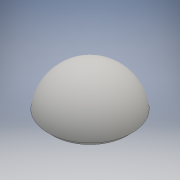
# Autodesk Inventor part: Part2
Saved by Autodesk Inventor 2016 (Build 200138000, 138)
## iProperties
Created: 2016-05-04
Part Number: Part2
Material: 一般
Document SubType Name: Modeling
Designer: 宏太
Density: 1 g/cm^3
Appearance: 既定
Author: 宏太
Autodesk Inventor part; units mm, degrees
ref_plane "YZ Plane" through (0, 0, 0) normal (1, 0, 0) x (0, 1, 0)
ref_plane "XZ Plane" through (0, 0, 0) normal (0, 1, 0) x (-1, 0, 0)
ref_plane "XY Plane" through (0, 0, 0) normal (0, 0, 1) x (1, 0, 0)
sketch "スケッチ1" plane through (0, 0, 0) normal (0, 1, 0) x (-1, 0, 0)
  arc A0 (22, 0) -> (0, 22) centre (0, 0) ccw
  line L0 (22, 0) -> (24.8364, 2.8551)
  arc A1 (24.8364, 2.8551) -> (0, 25) centre (0, 0) ccw
  line L1 (0, 25) -> (0, 22)
  point P0 (0, 0)
  dimension "d2" = 22
  constraints: 4 end point, 4 point on circle, 2 centre point, 1 vertical
  measures "d2" distance of point (0, 0) L0.start
revolve "回転1" add sketch "スケッチ1" angle 360 about axis through (0, 0, 25) along (0, 0, -1)
